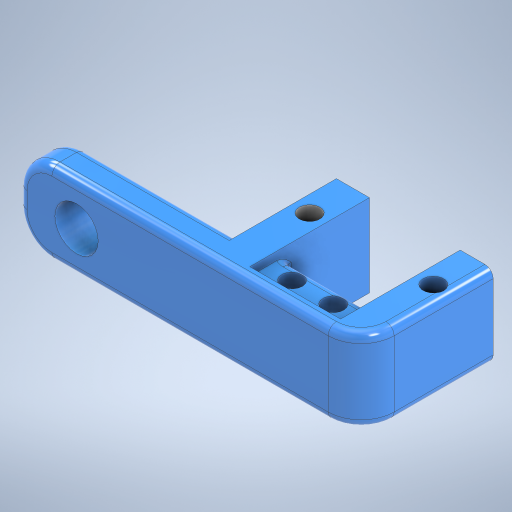
# Autodesk Inventor part: ServoMount
Saved by Autodesk Inventor 2024 (Build 280153000, 153)
## iProperties
Created: 2025-12-19
Part Number: ServoMount
Material: Generic
Document SubType Name: Modeling
Designer: Liam
Density: 1 g/cm^3
Appearance: Default
Mass: 16.9428 g
Surface Area: 79.0033 cm^2
Volume: 16.9428 cm^3
Author: Liam
Autodesk Inventor part; units mm, degrees
ref_plane "YZ Plane" through (0, 0, 0) normal (1, 0, 0) x (0, 1, 0)
ref_plane "XZ Plane" through (0, 0, 0) normal (0, 1, 0) x (-1, 0, 0)
sketch "Sketch1" plane through (0, 0, 0) normal (0, 1, 0) x (-1, 0, 0)
  line L0 (0, 0) -> (22, 0)
  line L1 (22, 0) -> (22, -42)
  line L2 (22, -42) -> (0, -42)
  line L3 (0, -42) -> (0, 0)
  circle A0 centre (6, 3.75) radius 2.5
  line L4 (22, -21) -> (0, -21) construction
  line L5 (30, -50) -> (30, 8)
  line L6 (30, 8) -> (-8, 8)
  line L7 (-8, 8) -> (-8, -50)
  line L8 (-8, -50) -> (30, -50)
  line L9 (11, 8) -> (11, 0) construction
  circle A1 centre (16, 3.75) radius 2.5
  circle A2 centre (6, -45.75) radius 2.5
  circle A3 centre (16, -45.75) radius 2.5
  line L10 (11, 0) -> (11, -42) construction
  line L11 (8, -42) -> (14, -42)
  line L12 (14, -42) -> (14, -45)
  line L13 (14, -45) -> (8, -45)
  line L14 (8, -45) -> (8, -42)
  circle A4 centre (-4, -10.5) radius 2.5
  circle A5 centre (26, -10.5) radius 2.5
  circle A6 centre (-4, -31.5) radius 2.5
  circle A7 centre (26, -31.5) radius 2.5
  line L15 (22, -21) -> (30, -21)
  line L16 (0, -21) -> (-8, -21)
  line L17 (30, 3) -> (75, 3)
  line L18 (75, 3) -> (75, 11)
  line L19 (75, 11) -> (30, 11)
  line L20 (30, 11) -> (30, 3)
  line L21 (30, 8) -> (-8, 8)
  line L22 (-8, 8) -> (-8, 11)
  line L23 (-8, 11) -> (30, 11)
  line L24 (30, 11) -> (30, 8)
  line L25 (22, 0) -> (22, 8)
  line L26 (0, 0) -> (0, 8)
  point P0 (30, 8)
  point P1 (30, 8)
  point P2 (30, 11)
  dimension "d0" = 42
  dimension "d1" = 22
  dimension "d7" = 5
  dimension "d12" = 8
  dimension "d13" = 58
  dimension "d14" = 38
  dimension "d15" = 3.75
  dimension "d16" = 5
  dimension "d17" = 49.5
  dimension "d31" = 4.25
  dimension "d32" = 6
  dimension "d33" = 3
  dimension "d34" = 3
  dimension "d35" = 5
  dimension "d36" = 4
  dimension "d37" = 10.5
  dimension "d40" = 30
  dimension "d43" = 21
  dimension "d51" = 8
  dimension "d52" = 3
  dimension "d53" = 45
  dimension "d97" = 38
  dimension "d98" = 3
  constraints: 54 end point, 10 parallel, 8 centre point, 7 midpoint, 7 perpendicular, 5 horizontal, 4 point on line, 3 symmetric about line, 1 vertical, 12 other
  measures "d0" distance of L2.end L0.start
  measures "d1" distance of L0.start L0.end
  measures "d7" diameter of A0
  measures "d12" distance between parallel lines of L1 L5
  measures "d13" distance of L6.end L7.end
  measures "d14" distance of L7.end L5.start
  measures "d15" distance from line of L0 A0.centre
  measures "d16" distance from line of L9 A0.centre
  measures "d17" distance of A2.centre A0.centre
  measures "d31" distance from line of L8 A2.centre
  measures "d32" distance of L12.end L13.end
  measures "d33" distance of L13.end L11.start
  measures "d34" distance between parallel lines of L10 L14
  measures "d35" diameter of A4
  measures "d36" distance from line of L3 A4.centre
  measures "d37" distance from line of L4 A4.centre
  measures "d40" distance of A4.centre A5.centre
  measures "d43" distance of A4.centre A6.centre
  measures "d51" distance of L17.end L18.end
  measures "d52" distance between parallel lines of L6 L19
  measures "d53" distance between parallel lines of L18 L20
  measures "d97" distance of L22.end L23.end
  measures "d98" distance of L21.end L22.end
extrude "Extrusion1" add sketch "Sketch1" along normal mid plane 20 contours L3 L16 L7 L6 L26 | L25 L6 L5 L15 L1 | L6 L22 L23 L20
extrude "Extrusion2" add sketch "Sketch1" along normal mid plane 20 contours L20 L19 L18 L17 L5
fillet "Fillet4" radius 8 3 edges at (8, 0, 11) (-75, 10, 7) (-75, -10, 7)
ref_plane "Work Plane3" through (0, 0, 2) normal (0, 0, 1) x (1, 0, 0)
sketch "Sketch5" plane through (0, 0, 2) normal (0, 0, 1) x (1, 0, 0)
  circle A0 centre (-61, 0) radius 5.25
  line L0 (-22, -10) -> (0, -10) projected
  point P0 (0, 0)
  point P1 (-11, -10)
  dimension "d112" = 10.5
  dimension "d143" = 50
  dimension "d147" = 10
  constraints: 1 centre point, 1 midpoint
  measures "d112" diameter of A0
  measures "d143" horizontal distance of point (-11, -10) A0.centre
  measures "d147" vertical distance of point (-11, -10) A0.centre
extrude "Extrusion6" cut sketch "Sketch5" along normal blind 10
extrude "Extrusion9" add sketch "Sketch1" along normal mid plane 16 contours L26 L6 L25 L0
fillet "Fillet11" radius 2 2 edges at (0, 0, 0) (-22, 0, 0)
fillet "Fillet12" radius 2 20 edges at (5.6569, 10, 8.6569) (8, 10, -9) (-72.6569, 7.6569, 11) (-75, 0, 11) (-72.6569, -7.6569, 11) (-33.5, -10, 11) (5.6569, -10, 8.6569) (8, -10, -9) (-33.5, 10, 11) (-72.6569, 7.6569, 3) (-75, 0, 3) (-72.6569, -7.6569, 3) (-48.5, -10, 3) (-48.5, 10, 3) (-11, 8, 0) (-0.5858, 8, -0.5858) (-21.4142, 8, -0.5858) (-0.5858, -8, -0.5858) (-21.4142, -8, -0.5858) (-11, -8, 0)
equation "\"d0\" = MOUNT_LENGTH"
equation "\"d1\" = MOUNT_WIDTH"
equation "\"d12\" = MOUNT_THICKNESS"
equation "\"d15\" = MOUNT_HOLE_Y"
equation "\"d16\" = MOUNT_HOLE_X"
equation "\"d36\" = 0.5 * MOUNT_THICKNESS"
equation "\"d37\" = 0.25 * MOUNT_LENGTH"
equation "\"d40\" = MOUNT_WIDTH + MOUNT_THICKNESS"
equation "\"d43\" = 0.5 * MOUNT_LENGTH"
equation "\"d51\" = COXA_HEIGHT"
equation "\"d53\" = COXA_LENGTH"
equation "\"d54\" = COXA_WIDTH"
equation "\"HoleDiameter\" = 3"
equation "\"InsertDiameter\" = 5"
equation "\"MOUNT_LENGTH\" = 42"
equation "\"MOUNT_WIDTH\" = 22"
equation "\"MOUNT_THICKNESS\" = 8"
equation "\"MOUNT_HOLE_Y\" = 3.75"
equation "\"MOUNT_HOLE_X\" = 5"
equation "\"COXA_HEIGHT\" = 8"
equation "\"COXA_LENGTH\" = 45"
equation "\"COXA_WIDTH\" = 20"
body "Solid1"
